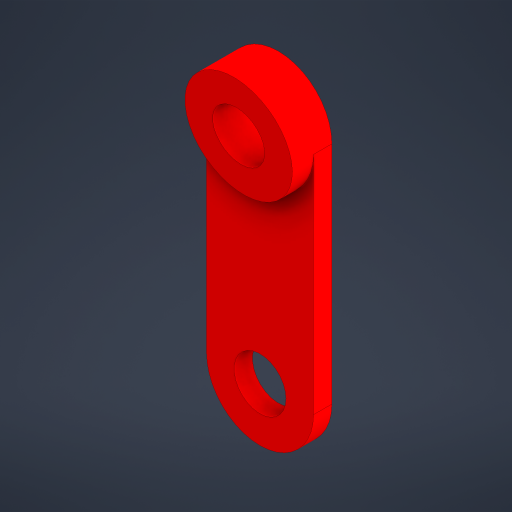
# Autodesk Inventor part: not flex back qre flex holder
Saved by Autodesk Inventor 2024 (Build 280153000, 153)
## iProperties
Created: 2024-03-06
Part Number: not flex back qre flex holder
Material: Všeobecné
Document SubType Name: Modeling
Designer: Simak
Density: 1 g/cm^3
Appearance: Výchozí
Author: Simak
Autodesk Inventor part; units mm, degrees
ref_plane "YZ Plane" through (0, 0, 0) normal (1, 0, 0) x (0, 1, 0)
ref_plane "XZ Plane" through (0, 0, 0) normal (0, 1, 0) x (-1, 0, 0)
ref_plane "XY Plane" through (0, 0, 0) normal (0, 0, 1) x (1, 0, 0)
sketch "Náčrt1" plane through (0, 0, 0) normal (0, 0, 1) x (1, 0, 0)
  line L0 (0, 7.375) -> (0, -7.375) construction
  line L1 (-3.5, 7.375) -> (-3.5, -7.375)
  line L2 (3.5, -7.375) -> (3.5, 7.375)
  arc A0 (3.5, 7.375) -> (-3.5, 7.375) centre (0, 7.375) ccw
  arc A1 (-3.5, -7.375) -> (3.5, -7.375) centre (0, -7.375) ccw
  circle A2 centre (0, 7.375) radius 1.7
  circle A3 centre (0, -7.375) radius 1.7
  circle A4 centre (0, 7.375) radius 3.5
  point P0 (0, 0)
  point P1 (0, 0)
  point P2 (-3.5, 7.375)
  point P3 (3.5, 7.375)
  dimension "d0" = 14.75
  dimension "d1" = 3.5
  dimension "d2" = 3.4
  constraints: 8 end point, 5 centre point, 4 coincident, 4 point on circle, 4 tangent, 2 equal radius, 1 midpoint, 1 parallel, 1 vertical
  measures "d0" distance of L0.end L0.start
  measures "d1" radius of A0
  measures "d2" diameter of A2
extrude "Vysunutí1" add sketch "Náčrt1" along normal blind 1.2
extrude "Vysunutí2" add sketch "Náčrt1" along normal blind 2.6 contours A0 A4
sketch "Náčrt4" plane through (3.5, -7.375, 0) normal (1, 0, 0) x (0, 0, -1)
  line L0 (-2.6, 13.05) -> (-2.6, 16.45) projected
  line L1 (-1.2, -1.7) -> (-1.2, 1.7) projected
  line L2 (-2.6, 14.75) -> (-1.2, 0)
  line L3 (-2.6, 18.25) -> (-2.6, 11.25) projected
  line L4 (0, 14.75) -> (0, 14.75) projected
  line L5 (0, 14.75) -> (-1.2, 14.75) projected
  line L6 (-1.2, 14.75) -> (-1.2, 14.75) projected
  line L7 (0, 14.75) -> (-1.2, 14.75) projected
  line L8 (-1.2, 11.25) -> (-2.6, 11.25) projected
  line L9 (-2.6, 14.75) -> (-2.9322, 18.25)
  line L10 (-2.6, 18.25) -> (-2.9322, 18.25)
  point P0 (0, 7.375)
  point P1 (-2.2678, 11.25)
  constraints: 6 end point, 2 midpoint, 1 collinear, 1 horizontal, 1 horizontal alignment
extrude "Vysunutí3" cut sketch "Náčrt4" against normal through all contours L0 L2 L8 L3
extrude "Vysunutí4" add sketch "Náčrt4" against normal up to surface (7 mm away) contours L9 L10 L3 L0
sketch "Náčrt5" plane through (0, 0, 0) normal (0, 0, -1) x (-1, 0, 0)
  circle A0 centre (0, 7.375) radius 1.7 projected
  circle A1 centre (0, -7.375) radius 1.7 projected
  line L0 (-3.5, -7.375) -> (-3.5, 7.375) projected
  arc A2 (-3.5, -7.375) -> (3.5, -7.375) centre (0, -7.375) ccw projected
  line L1 (3.5, 7.375) -> (3.5, -7.375) projected
  arc A3 (3.5, 7.375) -> (-3.5, 7.375) centre (0, 7.375) ccw projected
  arc A4 (1.7, 7.375) -> (-1.7, 7.375) centre (0, 7.375) ccw projected
  line L2 (-1.7, 7.375) -> (1.7, 7.375) projected
  arc A5 (3.5, 7.375) -> (0, 10.875) centre (0, 7.375) ccw projected
  line L3 (3.5, 10.875) -> (3.5, 7.375) projected
  line L4 (0, 10.875) -> (3.5, 10.875) projected
  arc A6 (0, 10.875) -> (-3.5, 7.375) centre (0, 7.375) ccw projected
  line L5 (-3.5, 10.875) -> (0, 10.875) projected
  line L6 (-3.5, 7.375) -> (-3.5, 10.875) projected
  point P0 (0, 0)
  point P1 (3.5, 7.375)
  point P2 (0, 10.875)
  point P3 (0, 10.875)
  point P4 (-3.5, 7.375)
  point P5 (-1.7, 7.375)
extrude "Vysunutí5" cut sketch "Náčrt5" against normal through all contours L2 A0 | L6 L5 A3 | L4 L3 A3 picked at (0.5018, 7.6383)
